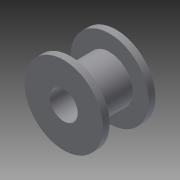
# Autodesk Inventor part: XcrLeftPulleyAlu
Saved by Autodesk Inventor 2013 (Build 170138000, 138)
## iProperties
Created: 2015-01-14
Part Number: XcrLeftPulleyAlu
Material: Generic
Document SubType Name: Modeling
Designer: dzban
Density: 1 g/cm^3
Author: dzban
Autodesk Inventor part; units mm, degrees
ref_plane "YZ Plane" through (0, 0, 0) normal (1, 0, 0) x (0, 1, 0)
ref_plane "XZ Plane" through (0, 0, 0) normal (0, 1, 0) x (-1, 0, 0)
ref_plane "XY Plane" through (0, 0, 0) normal (0, 0, 1) x (1, 0, 0)
sketch "Sketch1" plane through (0, 0, 0) normal (0, 0, 1) x (1, 0, 0)
  line L0 (2.5, 0) -> (2.5, 9.4)
  line L1 (2.5, 9.4) -> (7, 9.4)
  line L2 (7, 9.4) -> (7, 8.2)
  line L3 (7, 8.2) -> (4.15, 8.2)
  line L4 (4.15, 8.2) -> (4.15, 1.2)
  line L5 (4.15, 1.2) -> (7, 1.2)
  line L6 (7, 1.2) -> (7, 0)
  line L7 (7, 0) -> (2.5, 0)
  line L8 (0, 0) -> (0, 3.2914)
  dimension "d0" = 2.5
  dimension "d2" = 9.4
  dimension "d3" = 1.2
  dimension "d4" = 1.2
  dimension "d5" = 7
  dimension "d6" = 4.15
  constraints: 18 end point, 4 horizontal, 4 vertical, 1 collinear, 1 horizontal alignment
  measures "d0" distance between parallel lines of L0 L8
  measures "d2" distance between parallel lines of L1 L7
  measures "d3" distance between parallel lines of L1 L3
  measures "d4" distance between parallel lines of L5 L7
  measures "d5" distance between parallel lines of L6 L8
  measures "d6" distance between parallel lines of L4 L8
revolve "Revolution1" add sketch "Sketch1" angle 360 about axis through (0, 0, 0) along (0, 1, 0)
body "Solid1"
